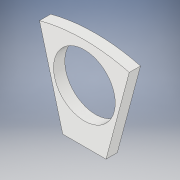
# Autodesk Inventor part: HA002
Saved by Autodesk Inventor 2017 SP1 (Build 210196100, 196)
## iProperties
Created: 2017-06-10
Part Number: HA002
Material: ABS Plastic
Document SubType Name: Modeling
Designer: Zach
Density: 1.06 g/cm^3
Appearance: CR White
Author: Zach
Autodesk Inventor part; units mm, degrees
ref_plane "YZ Plane" through (0, 0, 0) normal (1, 0, 0) x (0, 1, 0)
ref_plane "XZ Plane" through (0, 0, 0) normal (0, 1, 0) x (-1, 0, 0)
ref_plane "XY Plane" through (0, 0, 0) normal (0, 0, 1) x (1, 0, 0)
sketch "Sketch1" plane through (0, 0, 0) normal (0, 0, 1) x (1, 0, 0)
  line L0 (0, 0) -> (160, 0)
  line L1 (160, 0) -> (118.589, -154.5481)
  line L2 (0, 0) -> (41.411, -154.5481)
  line L3 (41.411, -154.5481) -> (118.589, -154.5481)
  dimension "d0" = 160
  dimension "d1" = 160
  dimension "d2" = 160
  dimension "d3" = 75
  dimension "d4" = 75
  constraints: 8 end point, 1 coincident, 1 horizontal
  measures "d0" distance of L0.start L0.end
  measures "d1" distance of L0.end L1.end
  measures "d2" distance of L0.start L2.end
  measures "d3" angle of L0 L1
  measures "d4" angle of L0 L2
extrude "Extrusion1" add sketch "Sketch1" along normal blind 20
sketch "Sketch5" plane through (0, 0, 20) normal (0, 0, 1) x (1, 0, 0)
  line L0 (160, 0) -> (0, 0) projected
  line L1 (160, 0) -> (256.5926, -25.8819)
  line L2 (118.589, -154.5481) -> (41.411, -154.5481) projected
  line L3 (118.589, -154.5481) -> (215.1815, -180.43)
  circle A0 centre (235.8871, -103.156) radius 80 construction
  arc A1 (215.1815, -180.43) -> (256.5926, -25.8819) centre (235.8871, -103.156) ccw
  line L4 (160, 0) -> (118.589, -154.5481)
  line L5 (0, 0) -> (41.411, -154.5481) projected
  line L6 (0, 0) -> (-96.5926, -25.8819)
  line L7 (41.411, -154.5481) -> (118.589, -154.5481) projected
  line L8 (41.411, -154.5481) -> (-55.1815, -180.43)
  circle A2 centre (-75.8871, -103.156) radius 80 construction
  arc A3 (-96.5926, -25.8819) -> (-55.1815, -180.43) centre (-75.8871, -103.156) ccw
  point P0 (90, 0)
  dimension "d25" = 100
  dimension "d26" = 100
  dimension "d27" = 160
  dimension "d30" = 100
  dimension "d31" = 100
  dimension "d32" = 160
  constraints: 10 end point, 8 point on circle, 6 tangent, 4 centre point, 1 concentric
  measures "d25" distance of L0.start L1.end
  measures "d26" distance of L2.start L3.end
  measures "d27" diameter of A0
  measures "d30" distance of L0.end L6.end
  measures "d31" distance of L2.end L8.end
  measures "d32" diameter of A2
extrude "Extrusion5" add sketch "Sketch5" against normal blind 20 contours L1 A1 L3 L4 | L5 L8 A3 L6
sketch "Sketch8" plane through (0, 0, 20) normal (0, 0, 1) x (1, 0, 0)
  line L0 (41.411, -154.5481) -> (118.589, -154.5481) projected
  line L1 (0, 0) -> (41.411, -154.5481)
  line L2 (0, 0) -> (160, 0) projected
  line L3 (160, 0) -> (118.589, -154.5481)
  line L4 (0, 0) -> (160, 0)
  line L5 (0, 0) -> (-96.5926, -25.8819) projected
  arc A0 (-96.5926, -25.8819) -> (-55.1815, -180.43) centre (-75.8871, -103.156) ccw projected
  line L6 (-55.1815, -180.43) -> (41.411, -154.5481) projected
  line L7 (215.1815, -180.43) -> (118.589, -154.5481) projected
  arc A1 (215.1815, -180.43) -> (256.5926, -25.8819) centre (235.8871, -103.156) ccw projected
  line L8 (160, 0) -> (256.5926, -25.8819) projected
  line L9 (160, 0) -> (0, 0) projected
  line L10 (160, 0) -> (256.5926, -25.8819) projected
  line L11 (0, 0) -> (160, 0)
  point P0 (90, 0)
  point P1 (70, 0)
  constraints: 8 end point, 1 collinear, 1 horizontal
extrude "Extrusion7" cut sketch "Sketch8" against normal through all contours L6 A0 L5 L1 | L3 L8 A1 L7
sketch "Sketch9" plane through (0, 0, 20) normal (0, 0, 1) x (1, 0, 0)
  circle A0 centre (80, -304.672) radius 315
  line L0 (0, 0) -> (160, 0)
  dimension "d37" = 630
  constraints: 2 end point, 2 point on circle, 1 centre point, 1 horizontal
  measures "d37" diameter of A0
extrude "Extrusion8" add sketch "Sketch9" against normal blind 20 contours L0 A0 picked at (60.8492, 1.6815)
sketch "Sketch10" plane through (0, 0, 20) normal (0, 0, 1) x (1, 0, 0)
  circle A0 centre (80, -60) radius 55
  line L0 (41.411, -154.5481) -> (118.589, -154.5481) projected
  point P0 (0, 0)
  point P1 (80, -154.5481)
  dimension "d40" = 110
  dimension "d41" = 60
  constraints: 1 centre point, 1 midpoint, 1 vertical alignment
  measures "d40" diameter of A0
  measures "d41" vertical distance of point (0, 0) A0.centre
extrude "Extrusion9" cut sketch "Sketch10" against normal through all
body "Solid1"
